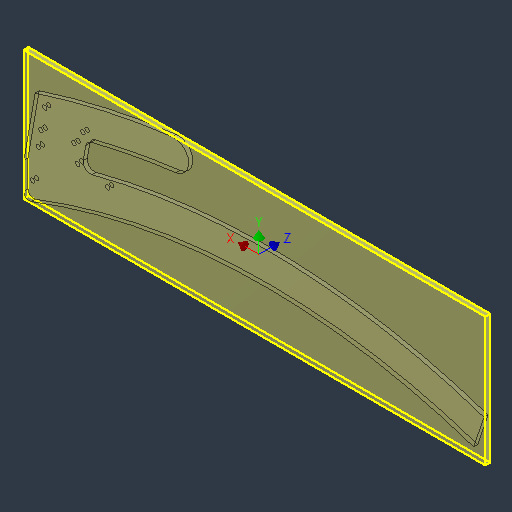
# Autodesk Inventor part: RACK,INSIDE
Saved by Autodesk Inventor 2026 (Build 300175050, 175E)
## iProperties
Created: 2026-04-01
Part Number: RACK,INSIDE
Material: Polycarbonate, PC 1000, Clear
Document SubType Name: Sheet Metal
Designer: 4aida
Density: 1.20131 g/cm^3
Sheet Metal Rule: Default
Appearance: Lexan (Clear)
Mass: 167.506 g
Surface Area: 664.034 cm^2
Volume: 139.436 cm^3
Author: 4aida
Autodesk Inventor part; units mm, degrees
ref_plane "YZ Plane" through (0, 0, 0) normal (1, 0, 0) x (0, 1, 0)
ref_plane "XZ Plane" through (0, 0, 0) normal (0, 1, 0) x (-1, 0, 0)
ref_plane "XY Plane" through (0, 0, 0) normal (0, 0, 1) x (1, 0, 0)
sketch "Sketch1" plane through (0, 0, 0) normal (0, 0, 1) x (1, 0, 0)
  line L0 (-282.4704, -20.4341) -> (-282.4704, 20.4341)
  line L1 (-394.804, 0) -> (382.9893, 0) construction
  arc A0 (245.5307, -6.7859) -> (-282.4704, -20.4341) centre (0, -728.1449) ccw
  arc A1 (257.8072, 29.282) -> (-282.4704, 20.4341) centre (0, -728.1449) ccw
  line L2 (245.5307, -6.7859) -> (257.8072, 29.282)
  line L3 (257.8072, 29.282) -> (259.8533, 35.2933)
  line L4 (259.8533, 35.2933) -> (271.8759, 31.2011)
  line L5 (271.8759, 31.2011) -> (255.5072, -16.8895)
  line L6 (255.5072, -16.8895) -> (243.4846, -12.7973)
  line L7 (243.4846, -12.7973) -> (245.5307, -6.7859)
  line L8 (0, 237.1551) -> (0, -889.0282) construction
  line L9 (0, -728.1449) -> (-282.4704, 0) construction
  arc A2 (205.7125, -1.0346) -> (-280.1164, -26.3317) centre (0, -728.1449) ccw
  line L10 (-280.1164, -26.3317) -> (-282.4704, -20.4341)
  line L11 (243.4846, -12.7973) -> (245.5307, -6.7859)
  point P0 (0, 0)
  point P1 (205.7125, -1.0346)
  dimension "d65" = 762
  dimension "d67" = 50.8
  dimension "d68" = 38.1
  dimension "d69" = 12.7
  dimension "d76" = 40
  dimension "d97" = 800.1
  dimension "d98" = 6.35
  measures "d65" radius of A0
  measures "d67" distance of L4.end L5.end
  measures "d68" radial gap between concentric circles of A1 A0
  measures "d69" distance of L3.end L4.end
  measures "d76" angle of L9 L2
  measures "d97" radius of A1
  measures "d98" radial gap between concentric circles of A0 A2
extrude "Plate1" add sketch "Sketch1" along normal blind 4.7625 contours L0 A1 L2 A0
sketch "Sketch3" plane through (0, 0, 0) normal (0, 0, -1) x (-1, 0, 0)
  line L0 (269.2384, 95.4765) -> (282.4704, 20.4341)
  arc A0 (282.4704, 20.4341) -> (-257.8072, 29.282) centre (0, -728.1449) ccw
  arc A1 (282.4704, -20.4341) -> (-245.5307, -6.7859) centre (0, -728.1449) ccw construction
  line L1 (0, -900.8528) -> (0, 308.1027) construction
  line L2 (-366.2845, 0) -> (393.0567, 0) construction
  arc A2 (269.2384, 95.4765) -> (108.3857, 131.5609) centre (0, -728.1449) ccw
  arc A3 (108.3857, 131.5609) -> (104.0502, 97.172) centre (106.218, 114.3664) ccw
  arc A4 (203.8267, 78.347) -> (104.0502, 97.172) centre (0, -728.1449) ccw
  arc A5 (209.7927, 71.9287) -> (203.8267, 78.347) centre (201.8507, 70.5283) ccw
  line L3 (209.7927, 71.9287) -> (212.772, 55.032)
  arc A6 (202.7861, 45.8305) -> (212.772, 55.032) centre (204.8301, 53.6316) ccw
  point P0 (0, 0)
  point P1 (-2.2036, 71.9521)
  dimension "d70" = 80
  dimension "d88" = 165.1
  dimension "d91" = 76.2
  dimension "d92" = 101.6
  dimension "d93" = 8.0645
  dimension "d95" = 31.75
  measures "d70" angle of L0 L2
  measures "d91" distance of L0.start L0.end
  measures "d93" radius of A6
  measures "d95" radial gap between concentric circles of A0 A4
sheet face with bend "Face2" sketch "Sketch3" thickness 4.7625 toward (0, 0, 1) bend radius 4.7625
bend "Bend1"
sketch "Sketch5" plane through (0, 0, 0) normal (0, 0, -1) x (-1, 0, 0)
  arc A0 (282.4704, -20.4341) -> (-245.5307, -6.7859) centre (0, -728.1449) ccw construction
  spline S0 degree 3 poles (-4.2317, 35.5309) (-3.9947, 36.2065) (-3.5205, 37.5578) (-2.7876, 39.577) (-2.0409, 41.5912) (-1.5294, 42.9288) (-1.2737, 43.5976) knots 0 0 0 0 0.214807 0.429614 0.644422 0.859229 0.859229 0.859229 0.859229
  spline S1 degree 3 poles (4.2317, 35.5309) (3.9947, 36.2065) (3.5205, 37.5578) (2.7876, 39.577) (2.0409, 41.5912) (1.5294, 42.9288) (1.2737, 43.5976) knots 0 0 0 0 0.214807 0.429614 0.644422 0.859229 0.859229 0.859229 0.859229
  circle A1 centre (0, -728.1449) radius 763.6875
  arc A2 (1.2737, 43.5976) -> (-1.2737, 43.5976) centre (0, -728.1449) ccw
  point P0 (-3.5169, 37.5565)
  point P1 (-2.7853, 39.5762)
  point P2 (-2.0375, 41.5899)
  point P3 (3.5169, 37.5565)
  point P4 (2.7853, 39.5762)
  point P5 (2.0375, 41.5899)
  constraints: 4 point on circle, 2 centre point, 22 other
extrude "Extrusion1" [suppressed]
pattern_circular "Circular Pattern1" [suppressed]
sketch "Sketch4" plane through (0, 0, 0) normal (0, 0, -1) x (-1, 0, 0)
  line L0 (282.4704, 20.4341) -> (269.2384, 95.4765) construction
  circle A0 centre (198.5568, 63.04) radius 25.4 construction
  line L1 (177.7503, 77.6089) -> (213.1256, 83.8465) construction
  line L2 (213.1256, 83.8465) -> (183.9879, 42.2336) construction
  line L3 (183.9879, 42.2336) -> (219.3632, 48.4712) construction
  line L4 (173.5426, 58.6294) -> (223.5709, 67.4507) construction
  line L5 (282.4704, 20.4341) -> (269.2384, 95.4765) construction
  line L6 (262.3523, 61.393) -> (265.6603, 42.6324) construction
  line L7 (0, -43.6162) -> (0, 118.6586) construction
  point P0 (0, 0)
  point P1 (257.9416, 86.4071)
  point P2 (272.2763, 5.1112)
  dimension "d31" = 25.4
  dimension "d33" = 12.7
  dimension "d34" = 12.7
  dimension "d42" = 50.8
  dimension "d43" = 45
  dimension "d51" = 5.2605
  dimension "d52" = 19.05
  dimension "d53" = 38.1
  dimension "d89" = 198.5568
  dimension "d90" = 63.04
  constraints: 10 end point, 9 coincident, 6 point on circle, 2 midpoint, 2 parallel, 2 point on line, 1 centre point, 1 perpendicular
  measures "d31" distance of L6.start point (257.942, 86.407)
  measures "d33" distance from line of L0 point (257.942, 86.407)
  measures "d34" distance from line of L0 L6.start
  measures "d42" diameter of A0
  measures "d43" angle of L1 L2
  measures "d51" distance from line of L1 point (257.942, 86.407)
  measures "d52" distance of L6.start L6.end
  measures "d53" distance of point (272.276, 5.111) point (265.66, 42.632)
  measures "d89" distance from line of L7 A0.centre
  measures "d90" vertical distance of A0.centre point (0, 0)
hole "Hole2" at (-257.9416, 86.4071, 0) at (-262.3523, 61.393, 0) at (-177.7503, 77.6089, 0) at (-173.5426, 58.6294, 0) at (-183.9879, 42.2336, 0) at (-219.3632, 48.4712, 0) at (-223.5709, 67.4507, 0) at (-213.1256, 83.8465, 0) at (-272.2763, 5.1112, 0) at (-265.6603, 42.6324, 0) direction (0, 0, 1) diameter 5.105 end through all clearance for "Flat Head Machine Screw (82)" size "#10" standard "Ansi Unified Screw Threads"
feature "Corner Round4" [suppressed]
feature "Corner Round5" [suppressed]
fillet "Corner Round6" radius 6.35 1 edges at (-282.4704, -20.4341, 2.3813)
equation "\"d33\" = d32"
equation "\"d34\" = d32"
equation "\"d40\" = Thickness"
equation "\"d5\" = Thickness"
equation "\"d22\" = BendRadius"
equation "\"d23\" = BendReliefWidth"
equation "\"d25\" = MinimumRemnant"
equation "\"d24\" = BendReliefDepth"
equation "\"d26\" = TransitionRadius"
equation "\"BendRadius\" = Thickness"
equation "\"BendReliefWidth\" = Thickness"
equation "\"BendReliefDepth\" = 0.5 * Thickness"
equation "\"CornerReliefSize\" = 4 * Thickness"
equation "\"MinimumRemnant\" = 2 * Thickness"
equation "\"TransitionRadius\" = BendRadius"
equation "\"JacobiRadiusSize\" = BendRadius"
equation "\"GapSize\" = Thickness"
equation "\"d32\" = 12.7"
equation "\"Thickness\" = 4.7625"
body "Solid1"
